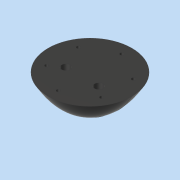
# Autodesk Inventor part: foreHullUpper
Saved by Autodesk Inventor 2017 (Build 210142000, 142)
## iProperties
Created: 2016-09-09
Part Number: foreHullUpper
Material: Polycarbonate, Clear
Document SubType Name: Modeling
Designer: techn
Density: 1.2 g/cm^3
Appearance: Smooth - Black
Mass: 764.223 g
Surface Area: 456.432 cm^2
Volume: 764.223 cm^3
Author: techn
Autodesk Inventor part; units mm, degrees
ref_plane "YZ Plane" through (0, 0, 0) normal (1, 0, 0) x (0, 1, 0)
ref_plane "XZ Plane" through (0, 0, 0) normal (0, 1, 0) x (-1, 0, 0)
sketch "Sketch6" plane through (0, 0, 0) normal (0, 0, 1) x (1, 0, 0)
  line L0 (540.6478, 1219.1491) -> (540.6478, -58.7076) construction
  line L1 (540.6478, -58.7076) -> (-407.4394, -58.7076) construction
  line L2 (-407.4394, -58.7076) -> (-407.4394, 1219.1491) construction
  line L3 (-407.4394, 1219.1491) -> (540.6478, 1219.1491) construction
  point P0 (0, 0)
  constraints: 2 other
sketch "Sketch5" plane through (0, 0, 0) normal (0, 0, 1) x (1, 0, 0)
  line L0 (0, 0) -> (0, 142.24)
  line L1 (0, 142.24) -> (50.8, 142.24)
  line L2 (50.8, 142.24) -> (-50.8, 142.24)
  line L3 (50.8, 142.24) -> (45.2986, 0) construction
  line L4 (45.2986, 0) -> (0, 0) construction
  spline S0 degree 2 poles (50.8, 142.24) (45.2986, 0) (0, 0) knots 1 1 1 2 2 2
  line L5 (-50.8, 142.24) -> (-45.2986, 0) construction
  line L6 (-45.2986, 0) -> (0, 0) construction
  spline S1 degree 2 poles (-50.8, 142.24) (-45.2986, 0) (0, 0) knots 1 1 1 2 2 2
  dimension "d20" = 142.24
  dimension "d21" = 50.8
  dimension "d22" = 101.6
  constraints: 6 end point, 1 horizontal, 1 perpendicular, 1 point on line, 1 symmetric about line, 1 vertical, 6 other
  measures "d20" distance of L0.start L0.end
  measures "d21" distance of L0.end L1.end
  measures "d22" distance of L1.end L2.end
revolve "Revolution1" add sketch "Sketch5" angle 360 about axis through (0, 0, 0) along (0, 1, 0) contours L0 L1 S0
ref_plane "Work Plane1" through (0, 21.59, 0) normal (0, 1, 0) x (1, 0, 0)
sketch "Sketch9" plane through (0, 21.59, 0) normal (0, 1, 0) x (1, 0, 0)
  line L0 (-101.4531, 67.0538) -> (104.6936, 67.0538)
  line L1 (104.6936, 67.0538) -> (104.6936, -70.5436)
  line L2 (104.6936, -70.5436) -> (-101.4531, -70.5436)
  line L3 (-101.4531, -70.5436) -> (-101.4531, 67.0538)
  point P0 (0, 0)
  constraints: 8 end point, 2 parallel, 1 horizontal, 1 perpendicular
extrude "Extrusion2" cut sketch "Sketch9" along normal through all
sketch "Sketch10" plane through (0, 21.59, 0) normal (0, 1, 0) x (1, 0, 0)
  line L0 (0, 0) -> (0, 22.225)
  circle A0 centre (0, 22.225) radius 1.27
  circle A1 centre (-19.2474, 11.1125) radius 1.27
  circle A2 centre (-19.2474, -11.1125) radius 1.27
  circle A3 centre (0, -22.225) radius 1.27
  circle A4 centre (19.2474, -11.1125) radius 1.27
  circle A5 centre (19.2474, 11.1125) radius 1.27
  dimension "d75" = 22.225
  dimension "d76" = 2.54
  dimension "d79" = 360
  constraints: 6 centre point, 2 end point, 1 coincident, 1 vertical, 13 other
  measures "d75" distance of L0.start L0.end
  measures "d76" diameter of A0
extrude "Extrusion3" cut sketch "Sketch10" against normal blind 6.35
sketch "Sketch11" plane through (0, 21.59, 0) normal (0, 1, 0) x (1, 0, 0)
  line L0 (0, 0) -> (11.5101, -5.3673)
  line L1 (0, 0) -> (12.7, 0) construction
  line L2 (0, 0) -> (0, 4.6472)
  circle A0 centre (11.5101, -5.3673) radius 3
  circle A1 centre (-11.5101, -5.3673) radius 3
  dimension "d83" = 12.7
  dimension "d84" = 25
  dimension "d85" = 6
  constraints: 6 end point, 2 centre point, 1 coincident, 1 equal length, 1 horizontal, 1 symmetric about line, 1 vertical, 1 other
  measures "d83" distance of L0.start L0.end
  measures "d84" angle of L0 L1
  measures "d85" diameter of A0
extrude "Extrusion4" cut sketch "Sketch11" against normal blind 25.4
body "Solid1"
